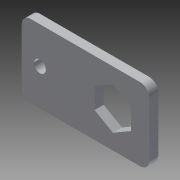
# Autodesk Inventor part: Hex Spacer 1-2
Saved by Autodesk Inventor 2014 (Build 180170000, 170)
## iProperties
Created: 2014-01-21
Part Number: Hex Spacer 1-2
Material: Aluminum 6061
Document SubType Name: Modeling
Designer: Michael
Density: 2.71 g/cm^3
Appearance: Aluminum - Flat
Author: Michael
Autodesk Inventor part; units mm, degrees
ref_plane "YZ Plane" through (0, 0, 0) normal (1, 0, 0) x (0, 1, 0)
ref_plane "XZ Plane" through (0, 0, 0) normal (0, 1, 0) x (-1, 0, 0)
ref_plane "XY Plane" through (0, 0, 0) normal (0, 0, 1) x (1, 0, 0)
sketch "Sketch1" plane through (0, 0, 0) normal (0, 0, 1) x (1, 0, 0)
  line L0 (0, 0) -> (44.45, 0)
  line L1 (44.45, 0) -> (44.45, 25.4)
  line L2 (44.45, 25.4) -> (0, 25.4)
  line L3 (0, 25.4) -> (0, 0)
  circle A0 centre (6.35, 12.7) radius 2.0701
  line L4 (31.75, 20.0323) -> (38.1, 16.3662)
  line L5 (38.1, 16.3662) -> (38.1, 9.0338)
  line L6 (38.1, 9.0338) -> (31.75, 5.3677)
  line L7 (31.75, 5.3677) -> (25.4, 9.0338)
  line L8 (25.4, 9.0338) -> (25.4, 16.3662)
  line L9 (25.4, 16.3662) -> (31.75, 20.0323)
  point P0 (31.75, 12.7)
  dimension "d0" = 44.45
  dimension "d1" = 25.4
  dimension "d2" = 4.1402
  dimension "d3" = 12.7
  dimension "d4" = 6.35
  dimension "d5" = 25.4
  dimension "d6" = 12.7
  dimension "d7" = 12.7
  constraints: 20 end point, 2 parallel, 1 centre point, 1 horizontal, 1 perpendicular, 1 vertical, 13 other
  measures "d0" distance of L2.end L1.end
  measures "d1" distance of L1.end L0.end
  measures "d2" diameter of A0
  measures "d3" distance from line of L0 A0.centre
  measures "d4" distance from line of L3 A0.centre
  measures "d5" distance of point (31.75, 12.7) A0.centre
  measures "d6" distance between parallel lines of L8 L5
  measures "d7" distance from line of L0 point (31.75, 12.7)
extrude "Extrusion1" add sketch "Sketch1" along normal blind 3.175
fillet "Fillet1" radius 3.175 4 edges at (44.45, 25.4, 1.5875) (44.45, 0, 1.5875) (0, 25.4, 1.5875) (0, 0, 1.5875)
body "Solid1"
